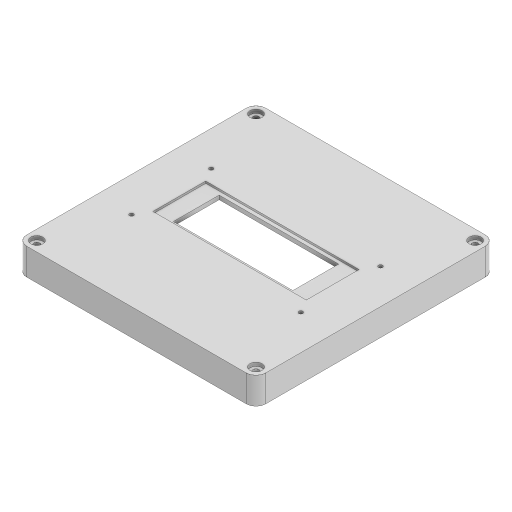
# Autodesk Inventor part: 3D printed box top
Saved by Autodesk Inventor 2023 (Build 270158000, 158)
## iProperties
Created: 2022-11-03
Part Number: 3D printed box top
Material: Generic
Document SubType Name: Modeling
Designer: ferrerx
Density: 1 g/cm^3
Appearance: Default
Author: ferrerx
Autodesk Inventor part; units mm, degrees
ref_plane "YZ Plane" through (0, 0, 0) normal (1, 0, 0) x (0, 1, 0)
ref_plane "XZ Plane" through (0, 0, 0) normal (0, 1, 0) x (-1, 0, 0)
ref_plane "XY Plane" through (0, 0, 0) normal (0, 0, 1) x (1, 0, 0)
sketch "Sketch1" plane through (0, 0, 0) normal (0, 1, 0) x (-1, 0, 0)
  line L0 (-55, 55) -> (55, 55)
  line L1 (55, 55) -> (55, -55)
  line L2 (55, -55) -> (-55, -55)
  line L3 (-55, -55) -> (-55, 55)
  line L4 (-55, 55) -> (55, -55) construction
  line L5 (55, 55) -> (-55, -55) construction
  line L6 (-12.5, 37.5) -> (12.5, 37.5) construction
  line L7 (12.5, 37.5) -> (12.5, -37.5) construction
  line L8 (12.5, -37.5) -> (-12.5, -37.5) construction
  line L9 (-12.5, -37.5) -> (-12.5, 37.5) construction
  line L10 (-12.5, 37.5) -> (12.5, -37.5) construction
  line L11 (12.5, 37.5) -> (-12.5, -37.5) construction
  line L12 (-37.5, 37.5) -> (37.5, 37.5) construction
  line L13 (37.5, 37.5) -> (37.5, -37.5) construction
  line L14 (37.5, -37.5) -> (-37.5, -37.5) construction
  line L15 (-37.5, -37.5) -> (-37.5, 37.5)
  line L16 (-37.5, 37.5) -> (37.5, -37.5) construction
  line L17 (37.5, 37.5) -> (-37.5, -37.5) construction
  circle A0 centre (37.5, -37.5) radius 2 construction
  circle A1 centre (37.5, 37.5) radius 2 construction
  circle A2 centre (-37.5, 37.5) radius 2 construction
  circle A3 centre (-37.5, -37.5) radius 2 construction
  point P0 (0, 0)
  dimension "d0" = 110
  dimension "d1" = 110
  dimension "d2" = 25
  dimension "d3" = 75
  dimension "d4" = 75
  dimension "d5" = 4
  dimension "d6" = 4
  dimension "d7" = 4
  dimension "d8" = 4
  constraints: 36 end point, 6 midpoint, 6 parallel, 4 centre point, 4 coincident, 3 horizontal, 3 perpendicular, 1 point on line
  measures "d0" distance of L1.end L2.end
  measures "d1" distance of L0.end L1.end
  measures "d2" distance of L7.end L8.end
  measures "d3" distance of L8.end L6.start
  measures "d4" distance of L13.end L14.end
  measures "d5" diameter of A0
  measures "d6" diameter of A1
  measures "d7" diameter of A2
  measures "d8" diameter of A3
extrude "Extrusion1" add sketch "Sketch1" along normal blind 3
sketch "Sketch3" plane through (0, 3, 0) normal (0, 1, 0) x (1, 0, 0)
  line L0 (35, -35) -> (-35, -35)
  line L1 (-35, -35) -> (-35, 35)
  line L2 (-35, 35) -> (35, 35)
  line L3 (35, 35) -> (35, -35)
  line L4 (35, -35) -> (-35, 35) construction
  line L5 (-35, -35) -> (35, 35) construction
  point P0 (0, 0)
  dimension "d18" = 70
  dimension "d19" = 70
  constraints: 12 end point, 2 midpoint, 2 parallel, 1 horizontal, 1 perpendicular
  measures "d18" distance of L1.end L2.end
  measures "d19" distance of L0.end L1.end
extrude "Extrusion3" [suppressed]
fillet "Fillet1" [suppressed]
sketch "Sketch4" plane through (0, 3, 0) normal (0, 1, 0) x (1, 0, 0)
  line L0 (28, -16) -> (42, -16)
  line L1 (42, -16) -> (42, 16)
  line L2 (42, 16) -> (28, 16)
  line L3 (28, 16) -> (28, -16)
  line L4 (28, -16) -> (42, 16) construction
  line L5 (42, -16) -> (28, 16) construction
  line L6 (35, 33) -> (35, -33) projected
  point P0 (0, 0)
  point P1 (35, 0)
  dimension "d23" = 14
  dimension "d24" = 32
  constraints: 12 end point, 3 midpoint, 2 parallel, 1 horizontal, 1 perpendicular
  measures "d23" distance of L1.end L2.end
  measures "d24" distance of L2.end L0.start
extrude "Extrusion4" [suppressed]
sketch "Sketch5" plane through (0, 3, 0) normal (0, 1, 0) x (1, 0, 0)
  line L0 (-30, -11.5) -> (30, -11.5)
  line L1 (30, -11.5) -> (30, 11.5)
  line L2 (30, 11.5) -> (-30, 11.5)
  line L3 (-30, 11.5) -> (-30, -11.5)
  line L4 (-30, -11.5) -> (30, 11.5) construction
  line L5 (30, -11.5) -> (-30, 11.5) construction
  point P0 (0, 0)
  dimension "d31" = 23
  dimension "d32" = 60
  constraints: 12 end point, 2 midpoint, 2 parallel, 1 horizontal, 1 perpendicular
  measures "d31" distance of L0.end L1.end
  measures "d32" distance of L0.start L0.end
extrude "Extrusion5" cut sketch "Sketch5" against normal blind 10
sketch "Sketch6" plane through (0, 3, 0) normal (0, 1, 0) x (1, 0, 0)
  line L0 (-38.5, 13.25) -> (38.5, 13.25)
  line L1 (38.5, 13.25) -> (38.5, -13.25)
  line L2 (38.5, -13.25) -> (-38.5, -13.25)
  line L3 (-38.5, -13.25) -> (-38.5, 13.25)
  line L4 (-38.5, 13.25) -> (38.5, -13.25) construction
  line L5 (38.5, 13.25) -> (-38.5, -13.25) construction
  point P0 (0, 0)
  dimension "d35" = 26.5
  dimension "d36" = 77
  constraints: 12 end point, 2 midpoint, 2 parallel, 1 horizontal, 1 perpendicular
  measures "d35" distance of L0.end L1.end
  measures "d36" distance of L0.start L0.end
extrude "Extrusion6" cut sketch "Sketch6" against normal blind 1
sketch "Sketch7" plane through (0, 3, 0) normal (0, 1, 0) x (1, 0, 0)
  line L0 (-42.5, -20) -> (42.5, -20) construction
  line L1 (42.5, -20) -> (42.5, 20) construction
  line L2 (42.5, 20) -> (-42.5, 20) construction
  line L3 (-42.5, 20) -> (-42.5, -20) construction
  line L4 (-42.5, -20) -> (42.5, 20) construction
  line L5 (42.5, -20) -> (-42.5, 20) construction
  circle A0 centre (-42.5, 20) radius 1
  circle A1 centre (42.5, 20) radius 1
  circle A2 centre (42.5, -20) radius 1
  circle A3 centre (-42.5, -20) radius 1
  point P0 (0, 0)
  dimension "d39" = 40
  dimension "d40" = 85
  dimension "d41" = 2
  dimension "d42" = 2
  dimension "d43" = 2
  dimension "d44" = 2
  constraints: 12 end point, 4 centre point, 4 coincident, 2 midpoint, 2 parallel, 1 horizontal, 1 perpendicular
  measures "d39" distance of L0.end L1.end
  measures "d40" distance of L0.start L0.end
  measures "d41" diameter of A0
  measures "d42" diameter of A1
  measures "d43" diameter of A3
  measures "d44" diameter of A2
extrude "Extrusion7" cut sketch "Sketch7" against normal through all
sketch "Sketch8" plane through (0, 3, 0) normal (0, 1, 0) x (1, 0, 0)
  line L0 (55, -55) -> (55, 55) projected
  line L1 (-55, 55) -> (55, 55)
  line L2 (55, 55) -> (55, -55)
  line L3 (55, -55) -> (-55, -55)
  line L4 (-55, -55) -> (-55, 55)
  line L5 (-55, 55) -> (55, -55) construction
  line L6 (55, 55) -> (-55, -55) construction
  line L7 (-60, 60) -> (60, 60)
  line L8 (60, 60) -> (60, -60)
  line L9 (60, -60) -> (-60, -60)
  line L10 (-60, -60) -> (-60, 60)
  line L11 (-60, 60) -> (60, -60) construction
  line L12 (60, 60) -> (-60, -60) construction
  point P0 (0, 0)
  dimension "d47" = 5
  constraints: 24 end point, 4 midpoint, 4 parallel, 2 horizontal, 2 perpendicular, 1 point on line
  measures "d47" distance between parallel lines of L8 L0
extrude "Extrusion8" add sketch "Sketch8" against normal blind 13.45
sketch "Sketch9" plane through (0, -10.45, 0) normal (0, -1, 0) x (1, 0, 0)
  line L0 (-55, 55) -> (55, 55) projected
  circle A0 centre (-55, 55) radius 3.5
  line L1 (55, 55) -> (55, -55) projected
  circle A1 centre (55, 55) radius 3.5
  line L2 (55, -55) -> (-55, -55) projected
  circle A2 centre (55, -55) radius 3.5
  circle A3 centre (-55, -55) radius 3.5
  point P0 (0, 0)
  dimension "d50" = 7
  dimension "d51" = 7
  dimension "d52" = 7
  dimension "d53" = 7
  constraints: 4 centre point, 3 coincident
  measures "d50" diameter of A1
  measures "d51" diameter of A2
  measures "d52" diameter of A3
  measures "d53" diameter of A0
extrude "Extrusion9" add sketch "Sketch9" against normal blind 13.45
fillet "Fillet3" radius 5 4 edges at (60, -3.725, -60) (60, -3.725, 60) (-60, -3.725, -60) (-60, -3.725, 60)
sketch "Sketch10" plane through (0, -10.45, 0) normal (0, -1, 0) x (1, 0, 0)
  arc A0 (-55, 51.5) -> (-51.5, 55) centre (-55, 55) ccw projected
  circle A1 centre (-55, 55) radius 1.45
  arc A2 (51.5, 55) -> (55, 51.5) centre (55, 55) ccw projected
  circle A3 centre (55, 55) radius 1.45
  arc A4 (55, -51.5) -> (51.5, -55) centre (55, -55) ccw projected
  circle A5 centre (55, -55) radius 1.45
  arc A6 (-51.5, -55) -> (-55, -51.5) centre (-55, -55) ccw projected
  circle A7 centre (-55, -55) radius 1.45
  point P0 (0, 0)
  dimension "d57" = 2.9
  dimension "d58" = 2.9
  dimension "d59" = 2.9
  dimension "d60" = 2.9
  constraints: 4 centre point, 4 coincident
  measures "d57" diameter of A1
  measures "d58" diameter of A3
  measures "d59" diameter of A7
  measures "d60" diameter of A5
extrude "Extrusion10" cut sketch "Sketch10" against normal blind 13.45
sketch "Sketch11" plane through (0, 3, 0) normal (0, 1, 0) x (1, 0, 0)
  circle A0 centre (-55, 55) radius 1.45 projected
  circle A1 centre (-55, 55) radius 3
  circle A2 centre (55, 55) radius 1.45 projected
  circle A3 centre (55, 55) radius 3
  circle A4 centre (55, -55) radius 1.45 projected
  circle A5 centre (55, -55) radius 3
  circle A6 centre (-55, -55) radius 1.45 projected
  circle A7 centre (-55, -55) radius 3
  point P0 (0, 0)
  dimension "d63" = 6
  dimension "d64" = 6
  dimension "d65" = 6
  dimension "d66" = 6
  constraints: 4 centre point, 4 coincident
  measures "d63" diameter of A5
  measures "d64" diameter of A7
  measures "d65" diameter of A3
  measures "d66" diameter of A1
extrude "Extrusion11" cut sketch "Sketch11" against normal blind 1.8 contours A0 | A1 | A2 | A3 | A5 | A7
body "Solid1"
